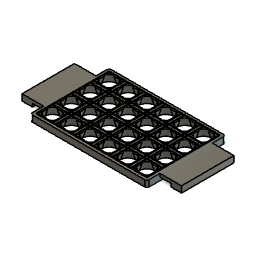
24_well_plate_adapter (Autodesk Fusion 360 design; units mm, degrees)
Autodesk Fusion 360 part; units mm, degrees
note: some values were not read from the file. Set by a fixed rule: which face or edge a step refers to.
sketch "Sketch1" plane through (0, 0, 0) normal (0, 1, 0) x (1, 0, 0)
  line L0 (0, 0) -> (130, 0)
  line L1 (130, 0) -> (130, -85)
  line L2 (130, -85) -> (0, -85)
  line L3 (0, -85) -> (0, 0)
  dimension "d1" = 130
  dimension "d2" = 85
  constraint horizontal L0
  constraint vertical L1
  constraint horizontal L2
  constraint vertical L3
  constraint coincident L0.start L3.end
  measures "d1" distance of L0.start L0.end
  measures "d2" distance of L0.start L2.end
extrude "Extrude1" add sketch "Sketch1" along normal blind 6 makes body 1
sketch "Sketch2" plane through (0, 6, 0) normal (0, 1, 0) x (-1, 0, 0)
  line L0 (0, 85) -> (-130, 85)
  line L1 (-130, 85) -> (-130, 0)
  line L2 (-130, 0) -> (0, 0)
  line L3 (0, 0) -> (0, 85)
  circle A0 centre (-20, 15) radius 7.75
  dimension "d5" = 15.5
  measures "d5" diameter of A0
extrude "Extrude2" cut sketch "Sketch2" against normal blind 6 contours A0 bodies 1
pattern_linear "R-Pattern1" count 6 spacing 18 along (1, 0, 0) count 4 spacing 18 along (0, 0, 1) of "Extrude2"
sketch "Sketch3" plane through (0, 6, 0) normal (0, 1, 0) x (-1, 0, 0)
  circle A0 centre (-110, 69) radius 7.75
  circle A1 centre (-92, 69) radius 7.75
  circle A2 centre (-74, 69) radius 7.75
  circle A3 centre (-56, 69) radius 7.75
  circle A4 centre (-38, 69) radius 7.75
  circle A5 centre (-20, 69) radius 7.75
  circle A6 centre (-110, 51) radius 7.75
  circle A7 centre (-92, 51) radius 7.75
  circle A8 centre (-74, 51) radius 7.75
  circle A9 centre (-56, 51) radius 7.75
  circle A10 centre (-38, 51) radius 7.75
  circle A11 centre (-20, 51) radius 7.75
  circle A12 centre (-110, 33) radius 7.75
  circle A13 centre (-92, 33) radius 7.75
  circle A14 centre (-74, 33) radius 7.75
  circle A15 centre (-56, 33) radius 7.75
  circle A16 centre (-38, 33) radius 7.75
  circle A17 centre (-20, 33) radius 7.75
  circle A18 centre (-110, 15) radius 7.75
  circle A19 centre (-92, 15) radius 7.75
  circle A20 centre (-74, 15) radius 7.75
  circle A21 centre (-56, 15) radius 7.75
  circle A22 centre (-38, 15) radius 7.75
  circle A23 centre (-20, 15) radius 7.75
  line L0 (0, 85) -> (-130, 85)
  line L1 (-130, 85) -> (-130, 0)
  line L2 (-130, 0) -> (0, 0)
  line L3 (0, 0) -> (0, 85)
  line L4 (-9.5, 4.5) -> (-120.5, 4.5)
  line L5 (-120.5, 4.5) -> (-120.5, 79.5)
  line L6 (-120.5, 79.5) -> (-9.5, 79.5)
  line L7 (-9.5, 79.5) -> (-9.5, 4.5)
  dimension "d12" = 111
  dimension "d13" = 75
  constraint horizontal L4
  constraint vertical L5
  constraint horizontal L6
  constraint vertical L7
  measures "d12" distance of L4.start L4.end
  measures "d13" distance of L4.start L6.end
extrude "Extrude3" cut sketch "Sketch3" against normal blind 6 contours L0 L1 L2 L3 bodies 1
ref_plane "WorkPlane1" through (65, 16, 42) normal (0, 1, 0) x (0, 0, 1)
sketch "Sketch4" plane through (65, 16, 42) normal (0, 1, 0) x (1, 0, 0)
sketch "Sketch5" plane through (65, 16, 42) normal (0, 1, 0) x (1, 0, 0)
  line L0 (1.25, 37) -> (1.75, 37)
  line L1 (1.75, 37) -> (1.75, -36)
  line L2 (1.75, -36) -> (1.25, -36)
  line L3 (1.25, -36) -> (1.25, 37)
  dimension "d17" = 0.5
  dimension "d18" = 73
  constraint horizontal L0
  constraint vertical L1
  constraint horizontal L2
  constraint vertical L3
  measures "d17" distance of L0.start L0.end
  measures "d18" distance of L0.start L2.end
extrude "Extrude4" add sketch "Sketch5" along normal blind 1 separate body makes body 2
copy_body "CopyPasteBodies1" bodies 2 makes body 3
move_body "Move1" bodies 3 to x (1, 0, 0) y (0, 1, 0) z (0, 0, 1) at (-3, 0, 0)
copy_body "CopyPasteBodies2" bodies 2 3 makes body 4 makes body 5
move_body "Move2" bodies 4 5 to x (1, 0, 0) y (0, 1, 0) z (0, 0, 1) at (18, 0, 0)
copy_body "CopyPasteBodies3" bodies 2 3 makes body 6 makes body 7
move_body "Move3" bodies 6 7 to x (1, 0, 0) y (0, 1, 0) z (0, 0, 1) at (36, 0, 0)
copy_body "CopyPasteBodies4" bodies 2 3 makes body 8 makes body 9
move_body "Move4" bodies 8 9 to x (1, 0, 0) y (0, 1, 0) z (0, 0, 1) at (-18, 0, 0)
copy_body "CopyPasteBodies5" bodies 2 3 makes body 10 makes body 11
move_body "Move5" bodies 10 11 to x (1, 0, 0) y (0, 1, 0) z (0, 0, 1) at (-36, 0, 0)
copy_body "CopyPasteBodies6" bodies 2 3 makes body 12 makes body 13
copy_body "CopyPasteBodies7" bodies 6 makes body 14
move_body "Move6" bodies 14 to x (1, 0, 0) y (0, 1, 0) z (0, 0, 1) at (15, 0, 0)
copy_body "CopyPasteBodies8" bodies 11 makes body 15
move_body "Move7" bodies 15 to x (1, 0, 0) y (0, 1, 0) z (0, 0, 1) at (-15, 0, 0)
ref_plane "WorkPlane2" through (65, 21, 42) normal (0, 1, 0) x (0, 0, 1)
sketch "Sketch6" plane through (65, 21, 42) normal (0, 1, 0) x (1, 0, 0)
  line L0 (-55, 1.75) -> (55, 1.75)
  line L1 (55, 1.75) -> (55, 1.25)
  line L2 (55, 1.25) -> (-55, 1.25)
  line L3 (-55, 1.25) -> (-55, 1.75)
  dimension "d22" = 110
  dimension "d23" = 0.5
  constraint horizontal L0
  constraint vertical L1
  constraint horizontal L2
  constraint vertical L3
  measures "d22" distance of L0.start L0.end
  measures "d23" distance of L0.start L2.end
extrude "Extrude5" add sketch "Sketch6" along normal blind 1 separate body makes body 16
copy_body "CopyPasteBodies9" bodies 16 makes body 17
move_body "Move8" bodies 17 to x (1, 0, 0) y (0, 1, 0) z (0, 0, 1) at (0, 0, 3)
copy_body "CopyPasteBodies10" bodies 16 17 makes body 18 makes body 19
move_body "Move9" bodies 18 19 to x (1, 0, 0) y (0, 1, 0) z (0, 0, 1) at (0, 0, 18)
copy_body "CopyPasteBodies11" bodies 16 17 makes body 20 makes body 21
move_body "Move10" bodies 20 21 to x (1, 0, 0) y (0, 1, 0) z (0, 0, 1) at (0, 0, -18)
copy_body "CopyPasteBodies12" bodies 20 makes body 22
move_body "Move11" bodies 22 to x (1, 0, 0) y (0, 1, 0) z (0, 0, 1) at (0, 0, -15)
copy_body "CopyPasteBodies13" bodies 19 makes body 23
move_body "Move12" bodies 23 to x (1, 0, 0) y (0, 1, 0) z (0, 0, 1) at (0, 0, 15)
move_body "Move13" bodies 23 22 21 20 19 18 17 16 to x (1, 0, 0) y (0, 1, 0) z (0, 0, 1) at (0, -5, 0)
combine "Combine1" operation add target body 23 tool bodies 22 21 20 19 17 18 16 15 14 13 12 11 10 9 8 7 6 5 4 3 2
sketch "Sketch7" plane through (65, 16, 42) normal (0, 1, 0) x (1, 0, 0)
  line L0 (-55, -36) -> (55, -36)
  line L1 (55, -36) -> (55, 37)
  line L2 (55, 37) -> (-55, 37)
  line L3 (-55, 37) -> (-55, -36)
  constraint horizontal L0
  constraint vertical L1
  constraint horizontal L2
  constraint vertical L3
extrude "Extrude6" add sketch "Sketch7" against normal blind 5.5 bodies 23
extrude "Extrude7" cut 24 faces at (17.5833, 16, 17.4167) (35.5833, 16, 17.4167) (53.5833, 16, 17.4167) (71.5833, 16, 17.4167) (89.5833, 16, 17.4167) (107.5833, 16, 17.4167) (107.5833, 16, 35.4167) (89.5833, 16, 35.4167) (71.5833, 16, 35.4167) (53.5833, 16, 35.4167) (35.5833, 16, 35.4167) (17.5833, 16, 35.4167) (17.5833, 16, 48.5833) (35.5833, 16, 48.5833) (53.5833, 16, 48.5833) (71.5833, 16, 48.5833) (89.5833, 16, 48.5833) (107.5833, 16, 48.5833) (107.5833, 16, 71.4167) (89.5833, 16, 71.4167) (71.5833, 16, 71.4167) (53.5833, 16, 71.4167) (35.5833, 16, 71.4167) (17.5833, 16, 71.4167) along direction (0, -1, 0) blind 5.5 on bodies 23 bodies 23
chamfer "Chamfer1" distance 0.5 distance2 5 96 edges at (12.75, 10.5, 69) (20, 10.5, 76.25) (30.75, 10.5, 69) (38, 10.5, 76.25) (48.75, 10.5, 69) (56, 10.5, 76.25) (66.75, 10.5, 69) (74, 10.5, 76.25) (84.75, 10.5, 69) (92, 10.5, 76.25) (102.75, 10.5, 69) (110, 10.5, 76.25) (12.75, 10.5, 51) (20, 10.5, 58.25) (30.75, 10.5, 51) (38, 10.5, 58.25) (48.75, 10.5, 51) (56, 10.5, 58.25) (66.75, 10.5, 51) (74, 10.5, 58.25) (84.75, 10.5, 51) (92, 10.5, 58.25) (102.75, 10.5, 51) (110, 10.5, 58.25) (12.75, 10.5, 33) (20, 10.5, 40.25) (30.75, 10.5, 33) (38, 10.5, 40.25) (56, 10.5, 40.25) (48.75, 10.5, 33) (66.75, 10.5, 33) (74, 10.5, 40.25) (84.75, 10.5, 33) (92, 10.5, 40.25) (102.75, 10.5, 33) (110, 10.5, 40.25) (12.75, 10.5, 15) (20, 10.5, 22.25) (30.75, 10.5, 15) (38, 10.5, 22.25) (48.75, 10.5, 15) (56, 10.5, 22.25) (66.75, 10.5, 15) (74, 10.5, 22.25) (84.75, 10.5, 15) (92, 10.5, 22.25) (102.75, 10.5, 15) (110, 10.5, 22.25) (110, 10.5, 7.75) (117.25, 10.5, 15) (92, 10.5, 7.75) (99.25, 10.5, 15) (74, 10.5, 7.75) (81.25, 10.5, 15) (56, 10.5, 7.75) (63.25, 10.5, 15) (38, 10.5, 7.75) (45.25, 10.5, 15) (20, 10.5, 7.75) (27.25, 10.5, 15) (20, 10.5, 25.75) (27.25, 10.5, 33) (20, 10.5, 43.75) (27.25, 10.5, 51) (20, 10.5, 61.75) (27.25, 10.5, 69) (38, 10.5, 61.75) (45.25, 10.5, 69) (56, 10.5, 61.75) (63.25, 10.5, 69) (74, 10.5, 61.75) (81.25, 10.5, 69) (92, 10.5, 61.75) (99.25, 10.5, 69) (110, 10.5, 61.75) (117.25, 10.5, 69) (117.25, 10.5, 51) (110, 10.5, 43.75) (92, 10.5, 43.75) (99.25, 10.5, 51) (74, 10.5, 43.75) (81.25, 10.5, 51) (56, 10.5, 43.75) (63.25, 10.5, 51) (38, 10.5, 43.75) (45.25, 10.5, 51) (38, 10.5, 25.75) (45.25, 10.5, 33) (56, 10.5, 25.75) (63.25, 10.5, 33) (74, 10.5, 25.75) (81.25, 10.5, 33) (92, 10.5, 25.75) (99.25, 10.5, 33) (110, 10.5, 25.75) (117.25, 10.5, 33) measured on face at (28.4167, 10.5, 71.4167) measured on face at (28.4167, 10.5, 71.4167) measured on face at (28.4167, 10.5, 71.4167) measured on face at (28.4167, 10.5, 71.4167) measured on face at (28.4167, 10.5, 71.4167) measured on face at (28.4167, 10.5, 71.4167) measured on face at (28.4167, 10.5, 71.4167) measured on face at (28.4167, 10.5, 71.4167) measured on face at (28.4167, 10.5, 71.4167) measured on face at (28.4167, 10.5, 71.4167) measured on face at (28.4167, 10.5, 71.4167) measured on face at (28.4167, 10.5, 71.4167) measured on face at (28.4167, 10.5, 71.4167) measured on face at (28.4167, 10.5, 71.4167) measured on face at (28.4167, 10.5, 71.4167) measured on face at (28.4167, 10.5, 71.4167) measured on face at (28.4167, 10.5, 71.4167) measured on face at (28.4167, 10.5, 71.4167) measured on face at (28.4167, 10.5, 71.4167) measured on face at (28.4167, 10.5, 71.4167) measured on face at (28.4167, 10.5, 71.4167) measured on face at (28.4167, 10.5, 71.4167) measured on face at (28.4167, 10.5, 71.4167) measured on face at (28.4167, 10.5, 71.4167) measured on face at (28.4167, 10.5, 71.4167) measured on face at (28.4167, 10.5, 71.4167) measured on face at (28.4167, 10.5, 71.4167) measured on face at (28.4167, 10.5, 71.4167) measured on face at (28.4167, 10.5, 71.4167) measured on face at (28.4167, 10.5, 71.4167) measured on face at (28.4167, 10.5, 71.4167) measured on face at (28.4167, 10.5, 71.4167) measured on face at (28.4167, 10.5, 71.4167) measured on face at (28.4167, 10.5, 71.4167) measured on face at (28.4167, 10.5, 71.4167) measured on face at (28.4167, 10.5, 71.4167) measured on face at (28.4167, 10.5, 71.4167) measured on face at (28.4167, 10.5, 71.4167) measured on face at (28.4167, 10.5, 71.4167) measured on face at (28.4167, 10.5, 71.4167) measured on face at (28.4167, 10.5, 71.4167) measured on face at (28.4167, 10.5, 71.4167) measured on face at (28.4167, 10.5, 71.4167) measured on face at (28.4167, 10.5, 71.4167) measured on face at (28.4167, 10.5, 71.4167) measured on face at (28.4167, 10.5, 71.4167) measured on face at (28.4167, 10.5, 71.4167) measured on face at (28.4167, 10.5, 71.4167) measured on face at (28.4167, 10.5, 71.4167) measured on face at (28.4167, 10.5, 71.4167) measured on face at (28.4167, 10.5, 71.4167) measured on face at (28.4167, 10.5, 71.4167) measured on face at (28.4167, 10.5, 71.4167) measured on face at (28.4167, 10.5, 71.4167) measured on face at (28.4167, 10.5, 71.4167) measured on face at (28.4167, 10.5, 71.4167) measured on face at (28.4167, 10.5, 71.4167) measured on face at (28.4167, 10.5, 71.4167) measured on face at (28.4167, 10.5, 71.4167) measured on face at (28.4167, 10.5, 71.4167) measured on face at (28.4167, 10.5, 71.4167) measured on face at (28.4167, 10.5, 71.4167) measured on face at (28.4167, 10.5, 71.4167) measured on face at (28.4167, 10.5, 71.4167) measured on face at (28.4167, 10.5, 71.4167) measured on face at (28.4167, 10.5, 71.4167) measured on face at (28.4167, 10.5, 71.4167) measured on face at (28.4167, 10.5, 71.4167) measured on face at (28.4167, 10.5, 71.4167) measured on face at (28.4167, 10.5, 71.4167) measured on face at (28.4167, 10.5, 71.4167) measured on face at (28.4167, 10.5, 71.4167) measured on face at (28.4167, 10.5, 71.4167) measured on face at (28.4167, 10.5, 71.4167) measured on face at (28.4167, 10.5, 71.4167) measured on face at (28.4167, 10.5, 71.4167) measured on face at (28.4167, 10.5, 71.4167) measured on face at (28.4167, 10.5, 71.4167) measured on face at (28.4167, 10.5, 71.4167) measured on face at (28.4167, 10.5, 71.4167) measured on face at (28.4167, 10.5, 71.4167) measured on face at (28.4167, 10.5, 71.4167) measured on face at (28.4167, 10.5, 71.4167) measured on face at (28.4167, 10.5, 71.4167) measured on face at (28.4167, 10.5, 71.4167) measured on face at (28.4167, 10.5, 71.4167) measured on face at (28.4167, 10.5, 71.4167) measured on face at (28.4167, 10.5, 71.4167) measured on face at (28.4167, 10.5, 71.4167) measured on face at (28.4167, 10.5, 71.4167) measured on face at (28.4167, 10.5, 71.4167) measured on face at (28.4167, 10.5, 71.4167) measured on face at (28.4167, 10.5, 71.4167) measured on face at (28.4167, 10.5, 71.4167) measured on face at (28.4167, 10.5, 71.4167) measured on face at (28.4167, 10.5, 71.4167) on bodies 23
ref_plane "WorkPlane3" through (65, 17, 41.5) normal (0, 1, 0) x (0, 0, 1)
sketch "Sketch8" plane through (65, 17, 41.5) normal (0, 1, 0) x (1, 0, 0)
  line L0 (-52.75, 34.25) -> (52.75, 34.25)
  line L1 (52.75, 34.25) -> (52.75, -35.25)
  line L2 (52.75, -35.25) -> (-52.75, -35.25)
  line L3 (-52.75, -35.25) -> (-52.75, 34.25)
  line L4 (-55, 36.5) -> (55, 36.5)
  line L5 (55, 36.5) -> (55, -36.5)
  line L6 (55, -36.5) -> (-55, -36.5)
  line L7 (-55, -36.5) -> (-55, 36.5)
  constraint horizontal L0
  constraint vertical L1
  constraint horizontal L2
  constraint vertical L3
  constraint horizontal L4
  constraint vertical L5
  constraint horizontal L6
  constraint vertical L7
extrude "Extrude8" cut sketch "Sketch8" against normal blind 1 bodies 23
move_body "Move14" bodies 23 to x (1, 0, 0) y (0, 1, 0) z (0, 0, 1) at (0, -10.5, 0)
combine "Combine2" operation add target body 1 tool bodies 23
sketch "Sketch9" plane through (120.5, 0, 0) normal (1, 0, 0) x (0, 0, -1)
  line L0 (-4.5, 6) -> (-79.5, 6)
  line L1 (-79.5, 6) -> (-79.5, 0)
  line L2 (-79.5, 0) -> (-4.5, 0)
  line L3 (-4.5, 0) -> (-4.5, 6)
sketch "Sketch10" plane through (9.5, 0, 0) normal (-1, 0, 0) x (0, 0, 1)
  line L0 (79.5, 6) -> (4.5, 6)
  line L1 (4.5, 6) -> (4.5, 0)
  line L2 (4.5, 0) -> (79.5, 0)
  line L3 (79.5, 0) -> (79.5, 6)
  line L4 (17, 0) -> (67, 0)
  line L5 (67, 0) -> (67, 6)
  line L6 (67, 6) -> (17, 6)
  line L7 (17, 6) -> (17, 0)
  dimension "d35" = 50
  constraint horizontal L4
  constraint vertical L5
  constraint horizontal L6
  constraint vertical L7
  constraint coincident L2 L4.start
  measures "d35" distance of L4.start L4.end
extrude "Extrude9" add sketch "Sketch10" along normal blind 20.5 contours L0 L2 L4 L5 L6 L7 bodies 1
sketch "Sketch11" plane through (0, 0, 0) normal (0, -1, 0) x (1, 0, 0)
  arc A0 (20, 22.75) -> (12.25, 15) centre (20, 15) ccw
  arc A1 (27.75, 15) -> (20, 22.75) centre (20, 15) ccw
  arc A2 (20, 7.25) -> (27.75, 15) centre (20, 15) ccw
  arc A3 (12.25, 15) -> (20, 7.25) centre (20, 15) ccw
  arc A4 (84.25, 15) -> (92, 7.25) centre (92, 15) ccw
  arc A5 (92, 22.75) -> (84.25, 15) centre (92, 15) ccw
  arc A6 (99.75, 15) -> (92, 22.75) centre (92, 15) ccw
  arc A7 (92, 7.25) -> (99.75, 15) centre (92, 15) ccw
  arc A8 (84.25, 33) -> (92, 25.25) centre (92, 33) ccw
  arc A9 (92, 40.75) -> (84.25, 33) centre (92, 33) ccw
  arc A10 (99.75, 33) -> (92, 40.75) centre (92, 33) ccw
  arc A11 (92, 25.25) -> (99.75, 33) centre (92, 33) ccw
  arc A12 (84.25, 51) -> (92, 43.25) centre (92, 51) ccw
  arc A13 (92, 58.75) -> (84.25, 51) centre (92, 51) ccw
  arc A14 (99.75, 51) -> (92, 58.75) centre (92, 51) ccw
  arc A15 (92, 43.25) -> (99.75, 51) centre (92, 51) ccw
  arc A16 (84.25, 69) -> (92, 61.25) centre (92, 69) ccw
  arc A17 (92, 76.75) -> (84.25, 69) centre (92, 69) ccw
  arc A18 (99.75, 69) -> (92, 76.75) centre (92, 69) ccw
  arc A19 (92, 61.25) -> (99.75, 69) centre (92, 69) ccw
  arc A20 (74, 76.75) -> (66.25, 69) centre (74, 69) ccw
  arc A21 (81.75, 69) -> (74, 76.75) centre (74, 69) ccw
  arc A22 (74, 61.25) -> (81.75, 69) centre (74, 69) ccw
  arc A23 (66.25, 69) -> (74, 61.25) centre (74, 69) ccw
  arc A24 (74, 58.75) -> (66.25, 51) centre (74, 51) ccw
  arc A25 (81.75, 51) -> (74, 58.75) centre (74, 51) ccw
  arc A26 (74, 43.25) -> (81.75, 51) centre (74, 51) ccw
  arc A27 (66.25, 51) -> (74, 43.25) centre (74, 51) ccw
  arc A28 (74, 40.75) -> (66.25, 33) centre (74, 33) ccw
  arc A29 (81.75, 33) -> (74, 40.75) centre (74, 33) ccw
  arc A30 (74, 25.25) -> (81.75, 33) centre (74, 33) ccw
  arc A31 (66.25, 33) -> (74, 25.25) centre (74, 33) ccw
  arc A32 (74, 22.75) -> (66.25, 15) centre (74, 15) ccw
  arc A33 (81.75, 15) -> (74, 22.75) centre (74, 15) ccw
  arc A34 (74, 7.25) -> (81.75, 15) centre (74, 15) ccw
  arc A35 (66.25, 15) -> (74, 7.25) centre (74, 15) ccw
  arc A36 (102.25, 15) -> (110, 7.25) centre (110, 15) ccw
  arc A37 (110, 22.75) -> (102.25, 15) centre (110, 15) ccw
  arc A38 (117.75, 15) -> (110, 22.75) centre (110, 15) ccw
  arc A39 (110, 7.25) -> (117.75, 15) centre (110, 15) ccw
  arc A40 (102.25, 33) -> (110, 25.25) centre (110, 33) ccw
  arc A41 (110, 40.75) -> (102.25, 33) centre (110, 33) ccw
  arc A42 (117.75, 33) -> (110, 40.75) centre (110, 33) ccw
  arc A43 (110, 25.25) -> (117.75, 33) centre (110, 33) ccw
  arc A44 (102.25, 51) -> (110, 43.25) centre (110, 51) ccw
  arc A45 (110, 58.75) -> (102.25, 51) centre (110, 51) ccw
  arc A46 (117.75, 51) -> (110, 58.75) centre (110, 51) ccw
  arc A47 (110, 43.25) -> (117.75, 51) centre (110, 51) ccw
  arc A48 (102.25, 69) -> (110, 61.25) centre (110, 69) ccw
  arc A49 (110, 76.75) -> (102.25, 69) centre (110, 69) ccw
  arc A50 (117.75, 69) -> (110, 76.75) centre (110, 69) ccw
  arc A51 (110, 61.25) -> (117.75, 69) centre (110, 69) ccw
  arc A52 (56, 25.25) -> (63.75, 33) centre (56, 33) ccw
  arc A53 (48.25, 33) -> (56, 25.25) centre (56, 33) ccw
  arc A54 (56, 40.75) -> (48.25, 33) centre (56, 33) ccw
  arc A55 (63.75, 33) -> (56, 40.75) centre (56, 33) ccw
  arc A56 (48.25, 15) -> (56, 7.25) centre (56, 15) ccw
  arc A57 (56, 22.75) -> (48.25, 15) centre (56, 15) ccw
  arc A58 (63.75, 15) -> (56, 22.75) centre (56, 15) ccw
  arc A59 (56, 7.25) -> (63.75, 15) centre (56, 15) ccw
  arc A60 (48.25, 51) -> (56, 43.25) centre (56, 51) ccw
  arc A61 (56, 58.75) -> (48.25, 51) centre (56, 51) ccw
  arc A62 (63.75, 51) -> (56, 58.75) centre (56, 51) ccw
  arc A63 (56, 43.25) -> (63.75, 51) centre (56, 51) ccw
  arc A64 (48.25, 69) -> (56, 61.25) centre (56, 69) ccw
  arc A65 (56, 76.75) -> (48.25, 69) centre (56, 69) ccw
  arc A66 (63.75, 69) -> (56, 76.75) centre (56, 69) ccw
  arc A67 (56, 61.25) -> (63.75, 69) centre (56, 69) ccw
  arc A68 (38, 76.75) -> (30.25, 69) centre (38, 69) ccw
  arc A69 (45.75, 69) -> (38, 76.75) centre (38, 69) ccw
  arc A70 (38, 61.25) -> (45.75, 69) centre (38, 69) ccw
  arc A71 (30.25, 69) -> (38, 61.25) centre (38, 69) ccw
  arc A72 (38, 58.75) -> (30.25, 51) centre (38, 51) ccw
  arc A73 (45.75, 51) -> (38, 58.75) centre (38, 51) ccw
  arc A74 (38, 43.25) -> (45.75, 51) centre (38, 51) ccw
  arc A75 (30.25, 51) -> (38, 43.25) centre (38, 51) ccw
  arc A76 (38, 40.75) -> (30.25, 33) centre (38, 33) ccw
  arc A77 (45.75, 33) -> (38, 40.75) centre (38, 33) ccw
  arc A78 (38, 25.25) -> (45.75, 33) centre (38, 33) ccw
  arc A79 (30.25, 33) -> (38, 25.25) centre (38, 33) ccw
  arc A80 (38, 22.75) -> (30.25, 15) centre (38, 15) ccw
  arc A81 (45.75, 15) -> (38, 22.75) centre (38, 15) ccw
  arc A82 (38, 7.25) -> (45.75, 15) centre (38, 15) ccw
  arc A83 (30.25, 15) -> (38, 7.25) centre (38, 15) ccw
  arc A84 (20, 76.75) -> (12.25, 69) centre (20, 69) ccw
  arc A85 (27.75, 69) -> (20, 76.75) centre (20, 69) ccw
  arc A86 (20, 61.25) -> (27.75, 69) centre (20, 69) ccw
  arc A87 (12.25, 69) -> (20, 61.25) centre (20, 69) ccw
  arc A88 (20, 58.75) -> (12.25, 51) centre (20, 51) ccw
  arc A89 (27.75, 51) -> (20, 58.75) centre (20, 51) ccw
  arc A90 (20, 43.25) -> (27.75, 51) centre (20, 51) ccw
  arc A91 (12.25, 51) -> (20, 43.25) centre (20, 51) ccw
  arc A92 (20, 40.75) -> (12.25, 33) centre (20, 33) ccw
  arc A93 (27.75, 33) -> (20, 40.75) centre (20, 33) ccw
  arc A94 (20, 25.25) -> (27.75, 33) centre (20, 33) ccw
  arc A95 (12.25, 33) -> (20, 25.25) centre (20, 33) ccw
  line L0 (9.5, 79.5) -> (9.5, 67)
  line L1 (9.5, 67) -> (-11, 67)
  line L2 (-11, 67) -> (-11, 17)
  line L3 (-11, 17) -> (9.5, 17)
  line L4 (9.5, 17) -> (9.5, 4.5)
  line L5 (9.5, 4.5) -> (120.5, 4.5)
  line L6 (120.5, 4.5) -> (120.5, 79.5)
  line L7 (120.5, 79.5) -> (9.5, 79.5)
  line L8 (9.5, 67) -> (-1, 67)
  line L9 (-1, 67) -> (-1, 17)
  line L10 (-1, 17) -> (9.5, 17)
  line L11 (9.5, 17) -> (9.5, 67)
  dimension "d38" = 10.5
  dimension "d39" = 50
  constraint horizontal L8
  constraint vertical L9
  constraint horizontal L10
  constraint vertical L11
  constraint coincident L0.end L1.start
  measures "d38" distance of L0.end L8.end
  measures "d39" distance of L0.end L3.end
extrude "Extrude10" cut sketch "Sketch11" against normal blind 3 contours L1 L3 L8 L9 L10 L11 bodies 1
sketch "Sketch12" plane through (120.5, 3, 42) normal (1, 0, 0) x (0, 0, -1)
  line L0 (-25, -3) -> (25, -3)
  line L1 (25, -3) -> (25, 3)
  line L2 (25, 3) -> (-25, 3)
  line L3 (-25, 3) -> (-25, -3)
  dimension "d42" = 50
  dimension "d43" = 6
  constraint horizontal L0
  constraint vertical L1
  constraint horizontal L2
  constraint vertical L3
  measures "d42" distance of L0.start L0.end
  measures "d43" distance of L0.start L2.end
extrude "Extrude11" add sketch "Sketch12" along normal blind 20.5 bodies 1
sketch "Sketch13" plane through (0, 0, 0) normal (0, -1, 0) x (1, 0, 0)
  arc A0 (20, 22.75) -> (12.25, 15) centre (20, 15) ccw
  arc A1 (27.75, 15) -> (20, 22.75) centre (20, 15) ccw
  arc A2 (20, 7.25) -> (27.75, 15) centre (20, 15) ccw
  arc A3 (12.25, 15) -> (20, 7.25) centre (20, 15) ccw
  arc A4 (84.25, 15) -> (92, 7.25) centre (92, 15) ccw
  arc A5 (92, 22.75) -> (84.25, 15) centre (92, 15) ccw
  arc A6 (99.75, 15) -> (92, 22.75) centre (92, 15) ccw
  arc A7 (92, 7.25) -> (99.75, 15) centre (92, 15) ccw
  arc A8 (84.25, 33) -> (92, 25.25) centre (92, 33) ccw
  arc A9 (92, 40.75) -> (84.25, 33) centre (92, 33) ccw
  arc A10 (99.75, 33) -> (92, 40.75) centre (92, 33) ccw
  arc A11 (92, 25.25) -> (99.75, 33) centre (92, 33) ccw
  arc A12 (84.25, 51) -> (92, 43.25) centre (92, 51) ccw
  arc A13 (92, 58.75) -> (84.25, 51) centre (92, 51) ccw
  arc A14 (99.75, 51) -> (92, 58.75) centre (92, 51) ccw
  arc A15 (92, 43.25) -> (99.75, 51) centre (92, 51) ccw
  arc A16 (84.25, 69) -> (92, 61.25) centre (92, 69) ccw
  arc A17 (92, 76.75) -> (84.25, 69) centre (92, 69) ccw
  arc A18 (99.75, 69) -> (92, 76.75) centre (92, 69) ccw
  arc A19 (92, 61.25) -> (99.75, 69) centre (92, 69) ccw
  arc A20 (74, 76.75) -> (66.25, 69) centre (74, 69) ccw
  arc A21 (81.75, 69) -> (74, 76.75) centre (74, 69) ccw
  arc A22 (74, 61.25) -> (81.75, 69) centre (74, 69) ccw
  arc A23 (66.25, 69) -> (74, 61.25) centre (74, 69) ccw
  arc A24 (74, 58.75) -> (66.25, 51) centre (74, 51) ccw
  arc A25 (81.75, 51) -> (74, 58.75) centre (74, 51) ccw
  arc A26 (74, 43.25) -> (81.75, 51) centre (74, 51) ccw
  arc A27 (66.25, 51) -> (74, 43.25) centre (74, 51) ccw
  arc A28 (74, 40.75) -> (66.25, 33) centre (74, 33) ccw
  arc A29 (81.75, 33) -> (74, 40.75) centre (74, 33) ccw
  arc A30 (74, 25.25) -> (81.75, 33) centre (74, 33) ccw
  arc A31 (66.25, 33) -> (74, 25.25) centre (74, 33) ccw
  arc A32 (74, 22.75) -> (66.25, 15) centre (74, 15) ccw
  arc A33 (81.75, 15) -> (74, 22.75) centre (74, 15) ccw
  arc A34 (74, 7.25) -> (81.75, 15) centre (74, 15) ccw
  arc A35 (66.25, 15) -> (74, 7.25) centre (74, 15) ccw
  arc A36 (102.25, 15) -> (110, 7.25) centre (110, 15) ccw
  arc A37 (110, 22.75) -> (102.25, 15) centre (110, 15) ccw
  arc A38 (117.75, 15) -> (110, 22.75) centre (110, 15) ccw
  arc A39 (110, 7.25) -> (117.75, 15) centre (110, 15) ccw
  arc A40 (102.25, 33) -> (110, 25.25) centre (110, 33) ccw
  arc A41 (110, 40.75) -> (102.25, 33) centre (110, 33) ccw
  arc A42 (117.75, 33) -> (110, 40.75) centre (110, 33) ccw
  arc A43 (110, 25.25) -> (117.75, 33) centre (110, 33) ccw
  arc A44 (102.25, 51) -> (110, 43.25) centre (110, 51) ccw
  arc A45 (110, 58.75) -> (102.25, 51) centre (110, 51) ccw
  arc A46 (117.75, 51) -> (110, 58.75) centre (110, 51) ccw
  arc A47 (110, 43.25) -> (117.75, 51) centre (110, 51) ccw
  arc A48 (102.25, 69) -> (110, 61.25) centre (110, 69) ccw
  arc A49 (110, 76.75) -> (102.25, 69) centre (110, 69) ccw
  arc A50 (117.75, 69) -> (110, 76.75) centre (110, 69) ccw
  arc A51 (110, 61.25) -> (117.75, 69) centre (110, 69) ccw
  arc A52 (56, 25.25) -> (63.75, 33) centre (56, 33) ccw
  arc A53 (48.25, 33) -> (56, 25.25) centre (56, 33) ccw
  arc A54 (56, 40.75) -> (48.25, 33) centre (56, 33) ccw
  arc A55 (63.75, 33) -> (56, 40.75) centre (56, 33) ccw
  arc A56 (48.25, 15) -> (56, 7.25) centre (56, 15) ccw
  arc A57 (56, 22.75) -> (48.25, 15) centre (56, 15) ccw
  arc A58 (63.75, 15) -> (56, 22.75) centre (56, 15) ccw
  arc A59 (56, 7.25) -> (63.75, 15) centre (56, 15) ccw
  arc A60 (48.25, 51) -> (56, 43.25) centre (56, 51) ccw
  arc A61 (56, 58.75) -> (48.25, 51) centre (56, 51) ccw
  arc A62 (63.75, 51) -> (56, 58.75) centre (56, 51) ccw
  arc A63 (56, 43.25) -> (63.75, 51) centre (56, 51) ccw
  arc A64 (48.25, 69) -> (56, 61.25) centre (56, 69) ccw
  arc A65 (56, 76.75) -> (48.25, 69) centre (56, 69) ccw
  arc A66 (63.75, 69) -> (56, 76.75) centre (56, 69) ccw
  arc A67 (56, 61.25) -> (63.75, 69) centre (56, 69) ccw
  arc A68 (38, 76.75) -> (30.25, 69) centre (38, 69) ccw
  arc A69 (45.75, 69) -> (38, 76.75) centre (38, 69) ccw
  arc A70 (38, 61.25) -> (45.75, 69) centre (38, 69) ccw
  arc A71 (30.25, 69) -> (38, 61.25) centre (38, 69) ccw
  arc A72 (38, 58.75) -> (30.25, 51) centre (38, 51) ccw
  arc A73 (45.75, 51) -> (38, 58.75) centre (38, 51) ccw
  arc A74 (38, 43.25) -> (45.75, 51) centre (38, 51) ccw
  arc A75 (30.25, 51) -> (38, 43.25) centre (38, 51) ccw
  arc A76 (38, 40.75) -> (30.25, 33) centre (38, 33) ccw
  arc A77 (45.75, 33) -> (38, 40.75) centre (38, 33) ccw
  arc A78 (38, 25.25) -> (45.75, 33) centre (38, 33) ccw
  arc A79 (30.25, 33) -> (38, 25.25) centre (38, 33) ccw
  arc A80 (38, 22.75) -> (30.25, 15) centre (38, 15) ccw
  arc A81 (45.75, 15) -> (38, 22.75) centre (38, 15) ccw
  arc A82 (38, 7.25) -> (45.75, 15) centre (38, 15) ccw
  arc A83 (30.25, 15) -> (38, 7.25) centre (38, 15) ccw
  arc A84 (20, 76.75) -> (12.25, 69) centre (20, 69) ccw
  arc A85 (27.75, 69) -> (20, 76.75) centre (20, 69) ccw
  arc A86 (20, 61.25) -> (27.75, 69) centre (20, 69) ccw
  arc A87 (12.25, 69) -> (20, 61.25) centre (20, 69) ccw
  arc A88 (20, 58.75) -> (12.25, 51) centre (20, 51) ccw
  arc A89 (27.75, 51) -> (20, 58.75) centre (20, 51) ccw
  arc A90 (20, 43.25) -> (27.75, 51) centre (20, 51) ccw
  arc A91 (12.25, 51) -> (20, 43.25) centre (20, 51) ccw
  arc A92 (20, 40.75) -> (12.25, 33) centre (20, 33) ccw
  arc A93 (27.75, 33) -> (20, 40.75) centre (20, 33) ccw
  arc A94 (20, 25.25) -> (27.75, 33) centre (20, 33) ccw
  arc A95 (12.25, 33) -> (20, 25.25) centre (20, 33) ccw
  line L0 (9.5, 79.5) -> (9.5, 4.5)
  line L1 (9.5, 4.5) -> (120.5, 4.5)
  line L2 (120.5, 4.5) -> (120.5, 17)
  line L3 (120.5, 17) -> (141, 17)
  line L4 (141, 17) -> (141, 67)
  line L5 (141, 67) -> (120.5, 67)
  line L6 (120.5, 67) -> (120.5, 79.5)
  line L7 (120.5, 79.5) -> (9.5, 79.5)
  line L8 (120.5, 67) -> (131, 67)
  line L9 (131, 67) -> (131, 17)
  line L10 (131, 17) -> (120.5, 17)
  line L11 (120.5, 17) -> (120.5, 67)
  dimension "d46" = 10.5
  dimension "d47" = 50
  constraint horizontal L8
  constraint vertical L9
  constraint horizontal L10
  constraint vertical L11
  constraint coincident L5.end L6.start
  measures "d46" distance of L5.end L8.end
  measures "d47" distance of L5.end L2.end
extrude "Extrude12" cut sketch "Sketch13" against normal blind 3 contours L3 L5 L8 L9 L10 L11 bodies 1
fillet "Fillet1" radius 2 2 edges at (9.5, 3, 79.5) (9.5, 3, 4.5) on bodies 1
fillet "Fillet2" radius 2 2 edges at (120.5, 3, 79.5) (120.5, 3, 4.5) on bodies 1
